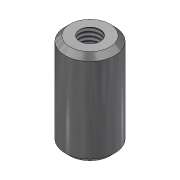
# Autodesk Inventor part: BC-10026
Saved by Autodesk Inventor 2016 (Build 200138000, 138)
## iProperties
Created: 2016-06-03
Part Number: BC-10026
Project: DIPOLO BC-3T- SIRIUS
Cost Center: 1504002005
Material: Aço Carbono VC131
Document SubType Name: Modeling
Designer: reinaldo.basilio
Density: 7.85 g/cm^3
Appearance: Semi-Polished
Mass: 10.2645 g
Surface Area: 8.90989 cm^2
Volume: 1.30758 cm^3
Description: Pino guia.
Stock Number: BC-10026
RuleStatus: InUse
DocNumber: XXXXX-XXX-XXXX-00-001.ipt
Folder: .
Title: DIPOLO BC-3T- SIRIUS
Author: reinaldo.basilio
Autodesk Inventor part; units mm, degrees
ref_plane "YZ Plane" through (0, 0, 0) normal (1, 0, 0) x (0, 1, 0)
ref_plane "XZ Plane" through (0, 0, 0) normal (0, 1, 0) x (-1, 0, 0)
ref_plane "XY Plane" through (0, 0, 0) normal (0, 0, 1) x (1, 0, 0)
sketch "Sketch5" plane through (0, 0, 0) normal (0, 0, 1) x (1, 0, 0)
  circle A0 centre (0, 0) radius 5
  dimension "d8" = 10
  constraints: 1 centre point, 1 coincident
  measures "d8" diameter of A0
extrude "Extrusion5" add sketch "Sketch5" along normal blind 19
hole "Hole2" at (0, 0, 19) direction (0, 0, -1) diameter 4.134 end through all thread size "M5x0.8" class "6H" standard "ANSI Metric M Profile"
chamfer "Chamfer1" distance 1 angle 45 2 edges at (-5, 0, 19) (-5, 0, 0)
body "Solid5"
